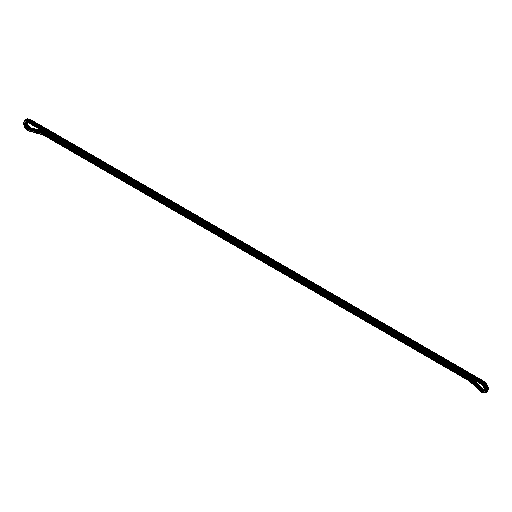
# Autodesk Inventor part: CHAIN
Saved by Autodesk Inventor 2022.5 (Build 265521000, 521)
## iProperties
Manager: 호상태
Company: 현대트랜시스(대유)
Created: 2023-01-26
Part Number: CHAIN
User Status: 2
Material: SCM435
Description: 3
Document SubType Name: Modeling
Designer: 박성규
Density: 7.84905 g/cm^3
Appearance: 후처리 없음
Project: SW-PJT
DETAIL: Coveryor Assembly
M/C TITLE: CJ 제일제당 협동로봇 포장시스탬 PILOT 장비
MAKER: HANKOOK CHAIN
PARTS NAME: Bracket
SPECIFICATION: TA20221101-CV200000-015
DocNumber: 221118_Standard_v1
Folder: .\
VDS_Category: 엔지니어링
Detail Description: Purchased products
Title: 2060VR x 426LINK
Subject: SW차종 시트조립라인
Author: 박성규
Revision Number: A
Autodesk Inventor part; units mm, degrees
ref_plane "YZ Plane" through (0, 0, 0) normal (1, 0, 0) x (0, 1, 0)
ref_plane "XZ Plane" through (0, 0, 0) normal (0, 1, 0) x (-1, 0, 0)
ref_plane "XY Plane" through (0, 0, 0) normal (0, 0, 1) x (1, 0, 0)
sketch "스케치9" plane through (0, 0, 0) normal (1, 0, 0) x (0, 1, 0)
  line L0 (-9.05, 0) -> (9.05, 0)
  line L1 (9.05, 0) -> (9.05, -7.75)
  line L2 (9.05, -7.75) -> (-9.05, -7.75)
  line L3 (-9.05, -7.75) -> (-9.05, 0)
  line L4 (-9.05, 0) -> (9.05, -7.75) construction
  line L5 (9.05, 0) -> (-9.05, -7.75) construction
  line L6 (-11.1, -7.75) -> (11.1, -7.75)
  line L7 (11.1, -7.75) -> (11.1, -16.25)
  line L8 (11.1, -16.25) -> (-11.1, -16.25)
  line L9 (-11.1, -16.25) -> (-11.1, -7.75)
  line L10 (-11.1, -7.75) -> (11.1, -16.25) construction
  line L11 (11.1, -7.75) -> (-11.1, -16.25) construction
  line L12 (-18, -16.25) -> (18, -16.25)
  line L13 (18, -16.25) -> (18, -31.25)
  line L14 (18, -31.25) -> (-18, -31.25)
  line L15 (-18, -31.25) -> (-18, -16.25)
  line L16 (-18, -16.25) -> (18, -31.25) construction
  line L17 (18, -16.25) -> (-18, -31.25) construction
  line L18 (-11.1, -31.25) -> (11.1, -31.25)
  line L19 (11.1, -31.25) -> (11.1, -39.75)
  line L20 (11.1, -39.75) -> (-11.1, -39.75)
  line L21 (-11.1, -39.75) -> (-11.1, -31.25)
  line L22 (-11.1, -31.25) -> (11.1, -39.75) construction
  line L23 (11.1, -31.25) -> (-11.1, -39.75) construction
  line L24 (-9.05, -39.75) -> (9.05, -39.75)
  line L25 (9.05, -39.75) -> (9.05, -47.5)
  line L26 (9.05, -47.5) -> (-9.05, -47.5)
  line L27 (-9.05, -47.5) -> (-9.05, -39.75)
  line L28 (-9.05, -39.75) -> (9.05, -47.5) construction
  line L29 (9.05, -39.75) -> (-9.05, -47.5) construction
  point P0 (0, 0)
  point P1 (0, -3.875)
  point P2 (0, -12)
  point P3 (0, -23.75)
  point P4 (0, -35.5)
  point P5 (0, -43.625)
  point P6 (0, -3.875)
  point P7 (0, -12)
  point P8 (0, -23.75)
  point P9 (0, -12)
  point P10 (0, -23.75)
  point P11 (0, -35.5)
  point P12 (0, -35.5)
  point P13 (0, -39.75)
  point P14 (0, 0)
  dimension "d38" = 7.75
  dimension "d39" = 8.5
  dimension "d40" = 15
  dimension "d41" = 8.5
  dimension "d42" = 7.75
  dimension "d43" = 18.1
  dimension "d44" = 22.2
  dimension "d45" = 36
  dimension "d46" = 47.5
  constraints: 60 end point, 19 midpoint, 10 parallel, 5 collinear, 5 horizontal, 5 perpendicular, 4 vertical alignment, 1 coincident, 1 point on line
  measures "d38" distance of L0.end L1.end
  measures "d39" distance of L6.end L7.end
  measures "d40" distance of L12.end L13.end
  measures "d41" distance of L18.end L19.end
  measures "d42" distance of L24.end L25.end
  measures "d43" distance of L0.start L0.end
  measures "d44" distance of L6.start L6.end
  measures "d45" distance of L12.start L12.end
  measures "d46" distance between parallel lines of L26 L0
sketch "스케치10" plane through (0, 0, 0) normal (0, 0, 1) x (1, 0, 0)
  circle A0 centre (0, -61.65) radius 61.65 construction
  circle A1 centre (-7910, -61.65) radius 61.65 construction
  circle A2 centre (-7640, -117.65) radius 61.65 construction
  circle A3 centre (-220, -117.65) radius 61.65 construction
  line L0 (-7910, 0) -> (0, 0)
  line L1 (-220, -56) -> (-7640, -56)
  line L2 (-200.3196, -59.2256) -> (-19.6804, -120.0744)
  line L3 (-7894.2065, -121.2427) -> (-7655.7935, -58.0573)
  arc A4 (-7910, 0) -> (-7894.2065, -121.2427) centre (-7910, -61.65) ccw
  arc A5 (-7640, -56) -> (-7655.7935, -58.0573) centre (-7640, -117.65) ccw
  arc A6 (-19.6804, -120.0744) -> (0, 0) centre (0, -61.65) ccw
  arc A7 (-200.3196, -59.2256) -> (-220, -56) centre (-220, -117.65) ccw
  dimension "d56" = 123.3
  dimension "d57" = 123.3
  dimension "d58" = 7910
  dimension "d59" = 123.3
  dimension "d60" = 123.3
  dimension "d62" = 220
  dimension "d63" = 56
  dimension "d64" = 270
  dimension "d65" = 56
  dimension "d68" = 246.6437
  dimension "d69" = 15.9716
  dimension "d70" = 7420
  dimension "d71" = 209.6508
  dimension "d72" = 190.6125
  constraints: 16 point on circle, 8 centre point, 8 end point, 6 tangent, 4 coincident, 1 horizontal, 1 horizontal alignment, 1 vertical alignment
  measures "d56" diameter of A0
  measures "d57" diameter of A1
  measures "d58" distance of A0.centre A1.centre
  measures "d59" diameter of A3
  measures "d60" diameter of A2
  measures "d62" horizontal distance of L0.end A3.centre
  measures "d63" vertical distance of A0.centre A3.centre
  measures "d64" horizontal distance of A2.centre A1.centre
  measures "d65" vertical distance of A1.centre A2.centre
  measures "d68" distance of L3.start L3.end
  measures "d70" distance of L1.start L1.end
  measures "d72" distance of L2.start L2.end
sweep "스윕2" add profiles "스케치9" path "스케치10" path curves L0 A4 L3 A5 L1 A7 L2 A6
equation "\"d41\" = d39"
equation "\"d42\" = d38"
equation "\"d57\" = d56"
equation "\"d59\" = d56"
equation "\"d60\" = d57"
equation "\"d65\" = d63"
equation "\"LINK\" = 0.0262467 * d70 + 0.0524934 * d69 + 0.0524934 * d71 + 0.0524934 * d68 + 0.0262467 * d58"
